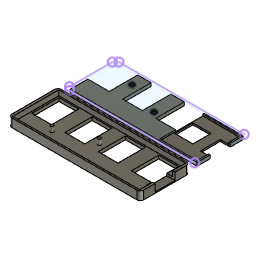
dongle_housing (Autodesk Fusion 360 design; units mm, degrees)
Autodesk Fusion 360 part; units mm, degrees
sketch "Sketch1" plane through (0, 0, 0) normal (0, 0, 1) x (1, 0, 0)
  line L0 (2, 0) -> (78, 0)
  line L1 (80, 2) -> (80, 28)
  line L2 (78, 30) -> (2, 30)
  line L3 (0, 28) -> (0, 2)
  arc A0 (2, 30) -> (0, 28) centre (2, 28) ccw
  arc A1 (0, 2) -> (2, 0) centre (2, 2) ccw
  arc A2 (80, 28) -> (78, 30) centre (78, 28) ccw
  arc A3 (78, 0) -> (80, 2) centre (78, 2) ccw
  point P0 (80, 0)
  point P1 (0, 30)
  dimension "d1" = 30
  dimension "d2" = 80
  dimension "d3" = 2
  dimension "d4" = 2
  dimension "d5" = 2
  dimension "d6" = 2
  constraint horizontal L0
  constraint vertical L1
  constraint horizontal L2
  constraint vertical L3
  constraint coincident P1 L2
  constraint coincident P1 L3
  constraint tangent L2 A0
  constraint tangent L3 A0
  constraint coincident origin L0
  constraint coincident origin L3
  constraint tangent L0 A1
  constraint tangent L3 A1
  constraint tangent L1 A2
  constraint tangent L2 A2
  constraint coincident P0 L0
  constraint coincident P0 L1
  constraint tangent L0 A3
  constraint tangent L1 A3
  measures "d1" distance of origin P1
  measures "d2" distance of origin P0
  measures "d3" radius of A0
  measures "d4" radius of A1
  measures "d5" radius of A2
  measures "d6" radius of A3
extrude "Extrude1" add sketch "Sketch1" along normal blind 6 makes body 1
sketch "Sketch2" plane through (0, 0, 6) normal (0, 0, 1) x (-1, 0, 0)
  arc A0 (-78, 0) -> (-80, -2) centre (-78, -2) ccw
  line L0 (-80, -2) -> (-80, -28)
  arc A1 (-80, -28) -> (-78, -30) centre (-78, -28) ccw
  line L1 (-78, -30) -> (-2, -30)
  arc A2 (-2, -30) -> (0, -28) centre (-2, -28) ccw
  line L2 (0, -28) -> (0, -2)
  arc A3 (0, -2) -> (-2, 0) centre (-2, -2) ccw
  line L3 (-2, 0) -> (-78, 0)
  line L4 (-40, -30) -> (-40, 0) construction
  line L5 (-2.5, -28.1) -> (-77.5, -28.1)
  line L6 (-77.5, -28.1) -> (-77.5, -1.9)
  line L7 (-77.5, -1.9) -> (-2.5, -1.9)
  line L8 (-2.5, -1.9) -> (-2.5, -28.1)
  line L9 (0, -15) -> (-80, -15) construction
  dimension "d11" = 75
  dimension "d12" = 26.2
  constraint midpoint L1 L4.start
  constraint midpoint L3 L4.end
  constraint horizontal L5
  constraint vertical L6
  constraint horizontal L7
  constraint vertical L8
  constraint symmetric L4 L6 L8
  constraint midpoint L2 L9.start
  constraint midpoint L0 L9.end
  constraint symmetric L5 L7 L9
  measures "d11" distance of L5.start L5.end
  measures "d12" distance of L5.end L6.end
extrude "Extrude2" cut sketch "Sketch2" against normal blind 4 contours L5 L6 L7 L8 bodies 1
sketch "Sketch4" plane through (0, 0, 6) normal (0, 0, 1) x (1, 0, 0)
  line L0 (2.5, 28.1) -> (14.5, 28.1)
  line L1 (14.5, 28.1) -> (14.5, 11.6)
  line L2 (14.5, 11.6) -> (2.5, 11.6)
  line L3 (2.5, 11.6) -> (2.5, 28.1)
  line L4 (34.6667, 28.1) -> (34.6667, 11.6)
  line L5 (22.6667, 28.1) -> (34.6667, 28.1)
  line L6 (22.6667, 11.6) -> (22.6667, 28.1)
  line L7 (34.6667, 11.6) -> (22.6667, 11.6)
  line L8 (54.8333, 28.1) -> (54.8333, 11.6)
  line L9 (42.8333, 28.1) -> (54.8333, 28.1)
  line L10 (42.8333, 11.6) -> (42.8333, 28.1)
  line L11 (54.8333, 11.6) -> (42.8333, 11.6)
  line L12 (75, 28.1) -> (75, 11.6)
  line L13 (63, 28.1) -> (75, 28.1)
  line L14 (63, 11.6) -> (63, 28.1)
  line L15 (75, 11.6) -> (63, 11.6)
  dimension "d23" = 16.5
  dimension "d24" = 12
  dimension "d27" = 60.5
  dimension "d28" = 0
  constraint horizontal L0
  constraint vertical L1
  constraint horizontal L2
  constraint vertical L3
  measures "d23" distance of L0.start L2.end
  measures "d24" distance of L0.start L0.end
extrude "Extrude4" cut sketch "Sketch4" against normal blind 11 bodies 1
sketch "Sketch5" plane through (0, 0, 6) normal (0, 0, 1) x (-1, 0, 0)
  line L0 (-77.5, -28.1) -> (-77.5, -1.9)
  line L1 (-77.5, -1.9) -> (-2.5, -1.9)
  line L2 (-2.5, -1.9) -> (-2.5, -28.1)
  line L3 (-2.5, -28.1) -> (-77.5, -28.1)
  arc A0 (-78, 0) -> (-80, -2) centre (-78, -2) ccw
  line L4 (-80, -2) -> (-80, -28)
  arc A1 (-80, -28) -> (-78, -30) centre (-78, -28) ccw
  line L5 (-78, -30) -> (-2, -30)
  arc A2 (-2, -30) -> (0, -28) centre (-2, -28) ccw
  line L6 (0, -28) -> (0, -2)
  arc A3 (0, -2) -> (-2, 0) centre (-2, -2) ccw
  line L7 (-2, 0) -> (-78, 0)
  line L8 (-80, -21.05) -> (-75, -21.05)
  line L9 (-75, -21.05) -> (-75, -8.95)
  line L10 (-75, -8.95) -> (-80, -8.95)
  line L11 (-80, -8.95) -> (-80, -21.05)
  line L12 (-80, -15) -> (0, -15) construction
  dimension "d31" = 12.1
  constraint horizontal L8
  constraint vertical L9
  constraint horizontal L10
  constraint vertical L11
  constraint coincident L4 L8.start
  constraint midpoint L4 L12.start
  constraint midpoint L6 L12.end
  constraint symmetric L8 L10 L12
  measures "d31" distance of L8.start L10.end
extrude "Extrude5" cut sketch "Sketch5" against normal blind 5.3 contours L0 L4 L8 L10 L11 | L0 L8 L9 L10 bodies 1
sketch "Sketch6" plane through (0, 0, 2) normal (0, 0, 1) x (-1, 0, 0)
  line L0 (-75, -8.95) -> (-75, -11.6)
  line L1 (-75, -11.6) -> (-63, -11.6)
  line L2 (-63, -11.6) -> (-63, -28.1)
  line L3 (-63, -28.1) -> (-54.8333, -28.1)
  line L4 (-54.8333, -28.1) -> (-54.8333, -11.6)
  line L5 (-54.8333, -11.6) -> (-42.8333, -11.6)
  line L6 (-42.8333, -11.6) -> (-42.8333, -28.1)
  line L7 (-42.8333, -28.1) -> (-34.6667, -28.1)
  line L8 (-34.6667, -28.1) -> (-34.6667, -11.6)
  line L9 (-34.6667, -11.6) -> (-22.6667, -11.6)
  line L10 (-22.6667, -11.6) -> (-22.6667, -28.1)
  line L11 (-22.6667, -28.1) -> (-14.5, -28.1)
  line L12 (-14.5, -28.1) -> (-14.5, -11.6)
  line L13 (-14.5, -11.6) -> (-2.5, -11.6)
  line L14 (-2.5, -11.6) -> (-2.5, -1.9)
  line L15 (-2.5, -1.9) -> (-77.5, -1.9)
  line L16 (-77.5, -1.9) -> (-77.5, -8.95)
  line L17 (-77.5, -8.95) -> (-75, -8.95)
  circle A0 centre (-18.17, -8.2) radius 0.95
  line L18 (-2, 0) -> (-78, 0)
  circle A1 centre (-39.2, -15.9) radius 0.95
  line L19 (-2.5, -1.9) -> (-2.5, -28.1)
  dimension "d34" = 15.67
  dimension "d35" = 8.2
  dimension "d36" = 1.9
  dimension "d37" = 12.2
  dimension "d38" = 36.7
  dimension "d39" = 1.9
  measures "d34" distance of L14 A0.centre
  measures "d35" distance of A0.centre L18
  measures "d36" diameter of A0
  measures "d37" distance of L7 A1.centre
  measures "d38" distance of A1.centre L19
  measures "d39" diameter of A1
extrude "Extrude6" add sketch "Sketch6" along normal blind 9.15 contours A0 | A1 bodies 1
sketch "Sketch7" plane through (0, 0, 0) normal (0, 0, 1) x (1, 0, 0)
  line L0 (2, 35) -> (78, 35)
  line L1 (80, 37) -> (80, 63)
  line L2 (78, 65) -> (2, 65)
  line L3 (0, 63) -> (0, 37)
  arc A0 (2, 65) -> (0, 63) centre (2, 63) ccw
  arc A1 (80, 63) -> (78, 65) centre (78, 63) ccw
  arc A2 (78, 35) -> (80, 37) centre (78, 37) ccw
  arc A3 (0, 37) -> (2, 35) centre (2, 37) ccw
  point P0 (0, 35)
  point P1 (80, 65)
  point P2 (0, 65)
  dimension "d42" = 30
  dimension "d43" = 80
  dimension "d44" = 2
  constraint horizontal L0
  constraint vertical L1
  constraint horizontal L2
  constraint vertical L3
  constraint coincident P2 L2
  constraint coincident P2 L3
  constraint tangent L2 A0
  constraint tangent L3 A0
  constraint coincident P1 L1
  constraint coincident P1 L2
  constraint tangent L1 A1
  constraint tangent L2 A1
  constraint equal A0 A1
  constraint tangent L0 A2
  constraint tangent L1 A2
  constraint equal A0 A2
  constraint coincident P0 L0
  constraint coincident P0 L3
  constraint tangent L0 A3
  constraint tangent L3 A3
  constraint equal A0 A3
  measures "d42" distance of P0 P2
  measures "d43" distance of P1 P2
  measures "d44" radius of A0
extrude "Extrude7" add sketch "Sketch7" along normal blind 4 separate body makes body 2
sketch "Sketch8" plane through (0, 0, 4) normal (0, 0, 1) x (-1, 0, 0)
  arc A0 (0, -37) -> (-2, -35) centre (-2, -37) ccw
  line L0 (-2, -35) -> (-78, -35)
  arc A1 (-78, -35) -> (-80, -37) centre (-78, -37) ccw
  line L1 (-80, -37) -> (-80, -63)
  arc A2 (-80, -63) -> (-78, -65) centre (-78, -63) ccw
  line L2 (-78, -65) -> (-2, -65)
  arc A3 (-2, -65) -> (0, -63) centre (-2, -63) ccw
  line L3 (0, -63) -> (0, -37)
  line L4 (-2.5, -36.9) -> (-77.5, -36.9)
  line L5 (-77.5, -36.9) -> (-77.5, -63.1)
  line L6 (-77.5, -63.1) -> (-2.5, -63.1)
  line L7 (-2.5, -63.1) -> (-2.5, -36.9)
  line L8 (-80, -50) -> (0, -50) construction
  line L9 (-40, -65) -> (-40, -35) construction
  dimension "d47" = 75
  dimension "d48" = 26.2
  dimension "d49" = 37.5
  dimension "d50" = 13.1
  constraint horizontal L4
  constraint vertical L5
  constraint horizontal L6
  constraint vertical L7
  constraint midpoint L1 L8.start
  constraint midpoint L3 L8.end
  constraint midpoint L2 L9.start
  constraint midpoint L0 L9.end
  measures "d47" distance of L5.end L6.end
  measures "d48" distance of L4 L6
  measures "d49" distance of L7 L9
  measures "d50" distance of L6 L8
extrude "Extrude8" cut sketch "Sketch8" against normal blind 2 contours L4 L5 L6 L7 bodies 2
sketch "Sketch9" plane through (0, 0, 2) normal (0, 0, 1) x (-1, 0, 0)
  line L0 (-2.5, -63.1) -> (-2.5, -36.9)
  line L1 (-2.5, -36.9) -> (-77.5, -36.9)
  line L2 (-77.5, -36.9) -> (-77.5, -63.1)
  line L3 (-77.5, -63.1) -> (-2.5, -63.1)
  line L4 (-2.5, -63.1) -> (-14.5, -63.1)
  line L5 (-14.5, -63.1) -> (-14.5, -46.6)
  line L6 (-14.5, -46.6) -> (-2.5, -46.6)
  line L7 (-2.5, -46.6) -> (-2.5, -63.1)
  line L8 (-34.65, -63.1) -> (-34.65, -46.6)
  line L9 (-22.65, -46.6) -> (-22.65, -63.1)
  line L10 (-34.65, -46.6) -> (-22.65, -46.6)
  line L11 (-22.65, -63.1) -> (-34.65, -63.1)
  line L12 (-54.8, -63.1) -> (-54.8, -46.6)
  line L13 (-42.8, -46.6) -> (-42.8, -63.1)
  line L14 (-54.8, -46.6) -> (-42.8, -46.6)
  line L15 (-42.8, -63.1) -> (-54.8, -63.1)
  dimension "d53" = 16.5
  dimension "d54" = 12
  dimension "d57" = -40.3
  dimension "d58" = 0
  constraint horizontal L4
  constraint vertical L5
  constraint horizontal L6
  constraint vertical L7
  constraint coincident L0.start L3.end
  measures "d53" distance of L0.start L6.end
  measures "d54" distance of L0.start L4.end
extrude "Extrude9" cut sketch "Sketch9" against normal blind 11 contours L0 L3 L4 L5 L6 L7 | L3 L8 L9 L10 L11 | L3 L12 L13 L14 L15 bodies 2
sketch "Sketch10" plane through (0, 0, 4) normal (0, 0, 1) x (-1, 0, 0)
  line L0 (-77.5, -36.9) -> (-2.5, -36.9)
  line L1 (-2.5, -36.9) -> (-2.5, -63.1)
  line L2 (-2.5, -63.1) -> (-77.5, -63.1)
  line L3 (-77.5, -63.1) -> (-77.5, -36.9)
  arc A0 (0, -37) -> (-2, -35) centre (-2, -37) ccw
  line L4 (-2, -35) -> (-78, -35)
  arc A1 (-78, -35) -> (-80, -37) centre (-78, -37) ccw
  line L5 (-80, -37) -> (-80, -63)
  arc A2 (-80, -63) -> (-78, -65) centre (-78, -63) ccw
  line L6 (-78, -65) -> (-2, -65)
  arc A3 (-2, -65) -> (0, -63) centre (-2, -63) ccw
  line L7 (0, -63) -> (0, -37)
  line L8 (-77.5, -43.95) -> (-83, -43.95)
  line L9 (-83, -43.95) -> (-83, -56.05)
  line L10 (-83, -56.05) -> (-77.5, -56.05)
  line L11 (-77.5, -56.05) -> (-77.5, -43.95)
  line L12 (-80, -50) -> (0, -50) construction
  line L13 (-77.5, -43.95) -> (-72.5, -43.95)
  line L14 (-72.5, -43.95) -> (-72.5, -56)
  line L15 (-72.5, -56) -> (-77.5, -56)
  line L16 (-77.5, -56) -> (-77.5, -43.95)
  dimension "d61" = 12.1
  dimension "d62" = 6.05
  dimension "d63" = 5
  constraint horizontal L8
  constraint vertical L9
  constraint horizontal L10
  constraint vertical L11
  constraint coincident L3 L8.start
  constraint midpoint L5 L12.start
  constraint midpoint L7 L12.end
  constraint horizontal L13
  constraint vertical L14
  constraint horizontal L15
  constraint vertical L16
  measures "d61" distance of L8.end L9.end
  measures "d62" distance of L10 L12
  measures "d63" distance of L8.start L13.end
extrude "Extrude10" cut sketch "Sketch10" against normal blind 2.5 contours L3 L11 L13 L14 L15 L16 | L3 L5 L8 L10 L11 L16 | L5 L8 L9 L10 bodies 2
sketch "Sketch11" plane through (0, 0, 2) normal (0, 0, 1) x (-1, 0, 0)
  line L0 (-72.5, -56) -> (-77.5, -56)
  line L1 (-77.5, -56) -> (-77.5, -56.05)
  line L2 (-77.5, -56.05) -> (-77.5, -63.1)
  line L3 (-77.5, -63.1) -> (-54.8, -63.1)
  line L4 (-54.8, -63.1) -> (-54.8, -46.6)
  line L5 (-54.8, -46.6) -> (-42.8, -46.6)
  line L6 (-42.8, -46.6) -> (-42.8, -63.1)
  line L7 (-42.8, -63.1) -> (-34.65, -63.1)
  line L8 (-34.65, -63.1) -> (-34.65, -46.6)
  line L9 (-34.65, -46.6) -> (-22.65, -46.6)
  line L10 (-22.65, -46.6) -> (-22.65, -63.1)
  line L11 (-22.65, -63.1) -> (-14.5, -63.1)
  line L12 (-14.5, -63.1) -> (-14.5, -46.6)
  line L13 (-14.5, -46.6) -> (-2.5, -46.6)
  line L14 (-2.5, -46.6) -> (-2.5, -36.9)
  line L15 (-2.5, -36.9) -> (-77.5, -36.9)
  line L16 (-77.5, -36.9) -> (-77.5, -43.95)
  line L17 (-77.5, -43.95) -> (-72.5, -43.95)
  line L18 (-72.5, -43.95) -> (-72.5, -56)
  line L19 (-77.5, -36.9) -> (-65.5, -36.9)
  line L20 (-65.5, -36.9) -> (-65.5, -63.1)
  line L21 (-65.5, -63.1) -> (-77.5, -63.1)
  line L22 (-77.5, -63.1) -> (-77.5, -36.9)
  dimension "d66" = 12
  constraint horizontal L19
  constraint vertical L20
  constraint horizontal L21
  constraint vertical L22
  constraint coincident L3 L20.end
  constraint coincident L15.end L16.start
  measures "d66" distance of L20 L22
extrude "Extrude11" cut sketch "Sketch11" against normal blind 1 contours L0 L1 L2 L3 L15 L16 L17 L18 L19 L20 L21 L22 bodies 2
sketch "Sketch12" plane through (0, 0, 2) normal (0, 0, 1) x (-1, 0, 0)
  line L0 (-65.5, -36.9) -> (-65.5, -63.1)
  line L1 (-65.5, -63.1) -> (-54.8, -63.1)
  line L2 (-54.8, -63.1) -> (-54.8, -46.6)
  line L3 (-54.8, -46.6) -> (-42.8, -46.6)
  line L4 (-42.8, -46.6) -> (-42.8, -63.1)
  line L5 (-42.8, -63.1) -> (-34.65, -63.1)
  line L6 (-34.65, -63.1) -> (-34.65, -46.6)
  line L7 (-34.65, -46.6) -> (-22.65, -46.6)
  line L8 (-22.65, -46.6) -> (-22.65, -63.1)
  line L9 (-22.65, -63.1) -> (-14.5, -63.1)
  line L10 (-14.5, -63.1) -> (-14.5, -46.6)
  line L11 (-14.5, -46.6) -> (-2.5, -46.6)
  line L12 (-2.5, -46.6) -> (-2.5, -36.9)
  line L13 (-2.5, -36.9) -> (-65.5, -36.9)
  line L14 (-55.5, -56.4) -> (-66.5, -56.4)
  line L15 (-66.5, -56.4) -> (-66.5, -45.4)
  line L16 (-66.5, -45.4) -> (-55.5, -45.4)
  line L17 (-55.5, -45.4) -> (-55.5, -56.4)
  line L18 (-77.5, -37) -> (-77.5, -63) construction
  dimension "d69" = 11
  dimension "d70" = 11
  dimension "d71" = 11
  dimension "d109" = 8.5
  constraint horizontal L14
  constraint vertical L15
  constraint horizontal L16
  constraint vertical L17
  constraint parallel L2 L18
  measures "d69" distance of L14.end L15.end
  measures "d70" distance of L14.start L14.end
  measures "d71" distance of L15 L18
  measures "d109" distance of L13 L16
extrude "Extrude12" cut sketch "Sketch12" against normal blind 8 contours L0 L14 L16 L17 | L0 L14 L15 L16 bodies 2
sketch "Sketch13" plane through (0, 0, 2) normal (0, 0, 1) x (-1, 0, 0)
  line L0 (-55.5, -56.4) -> (-65.5, -56.4)
  line L1 (-65.5, -56.4) -> (-65.5, -63.1)
  line L2 (-65.5, -63.1) -> (-54.8, -63.1)
  line L3 (-54.8, -63.1) -> (-54.8, -46.6)
  line L4 (-54.8, -46.6) -> (-42.8, -46.6)
  line L5 (-42.8, -46.6) -> (-42.8, -63.1)
  line L6 (-42.8, -63.1) -> (-34.65, -63.1)
  line L7 (-34.65, -63.1) -> (-34.65, -46.6)
  line L8 (-34.65, -46.6) -> (-22.65, -46.6)
  line L9 (-22.65, -46.6) -> (-22.65, -63.1)
  line L10 (-22.65, -63.1) -> (-14.5, -63.1)
  line L11 (-14.5, -63.1) -> (-14.5, -46.6)
  line L12 (-14.5, -46.6) -> (-2.5, -46.6)
  line L13 (-2.5, -46.6) -> (-2.5, -36.9)
  line L14 (-2.5, -36.9) -> (-65.5, -36.9)
  line L15 (-65.5, -36.9) -> (-65.5, -45.4)
  line L16 (-65.5, -45.4) -> (-55.5, -45.4)
  line L17 (-55.5, -45.4) -> (-55.5, -56.4)
  line L18 (-54.8, -63.1) -> (-65.5, -63.1)
  line L19 (-65.5, -63.1) -> (-65.5, -36.9)
  line L20 (-65.5, -36.9) -> (-54.8, -36.9)
  line L21 (-54.8, -36.9) -> (-54.8, -63.1)
  constraint horizontal L18
  constraint vertical L19
  constraint horizontal L20
  constraint vertical L21
  constraint coincident L14.end L15.start
  constraint coincident L2.end L3.start
extrude "Extrude13" cut sketch "Sketch13" against normal blind 1 contours L0 L1 L2 L3 L14 L15 L16 L17 L18 L19 L20 L21 bodies 2
sketch "Sketch14" plane through (0, 0, 6) normal (0, 0, 1) x (-1, 0, 0)
  line L0 (-77.5, -21.05) -> (-80, -21.05)
  line L1 (-80, -21.05) -> (-80, -28)
  arc A0 (-80, -28) -> (-78, -30) centre (-78, -28) ccw
  line L2 (-78, -30) -> (-2, -30)
  arc A1 (-2, -30) -> (0, -28) centre (-2, -28) ccw
  line L3 (0, -28) -> (0, -2)
  arc A2 (0, -2) -> (-2, 0) centre (-2, -2) ccw
  line L4 (-2, 0) -> (-78, 0)
  arc A3 (-78, 0) -> (-80, -2) centre (-78, -2) ccw
  line L5 (-80, -2) -> (-80, -8.95)
  line L6 (-80, -8.95) -> (-77.5, -8.95)
  line L7 (-77.5, -8.95) -> (-77.5, -1.9)
  line L8 (-77.5, -1.9) -> (-2.5, -1.9)
  line L9 (-2.5, -1.9) -> (-2.5, -28.1)
  line L10 (-2.5, -28.1) -> (-77.5, -28.1)
  line L11 (-77.5, -28.1) -> (-77.5, -21.05)
  line L12 (-1.5, -1) -> (-78.5, -1)
  line L13 (-78.5, -1) -> (-78.5, -29)
  line L14 (-78.5, -29) -> (-1.5, -29)
  line L15 (-1.5, -29) -> (-1.5, -1)
  dimension "d77" = 77
  dimension "d78" = 28
  dimension "d79" = 1
  dimension "d80" = 1.5
  constraint horizontal L12
  constraint vertical L13
  constraint horizontal L14
  constraint vertical L15
  measures "d77" distance of L12.start L12.end
  measures "d78" distance of L12.start L14.end
  measures "d79" distance of L4 L12
  measures "d80" distance of L3 L15
extrude "Extrude14" cut sketch "Sketch14" against normal blind 2.87 contours L0 L6 L7 L8 L9 L10 L11 L12 L13 L14 L15 bodies 1
sketch "Sketch15" plane through (0, 0, 4) normal (0, 0, 1) x (-1, 0, 0)
  line L0 (-77.5, -56.05) -> (-80, -56.05)
  line L1 (-80, -56.05) -> (-80, -63)
  arc A0 (-80, -63) -> (-78, -65) centre (-78, -63) ccw
  line L2 (-78, -65) -> (-2, -65)
  arc A1 (-2, -65) -> (0, -63) centre (-2, -63) ccw
  line L3 (0, -63) -> (0, -37)
  arc A2 (0, -37) -> (-2, -35) centre (-2, -37) ccw
  line L4 (-2, -35) -> (-78, -35)
  arc A3 (-78, -35) -> (-80, -37) centre (-78, -37) ccw
  line L5 (-80, -37) -> (-80, -43.95)
  line L6 (-80, -43.95) -> (-77.5, -43.95)
  line L7 (-77.5, -43.95) -> (-77.5, -36.9)
  line L8 (-77.5, -36.9) -> (-2.5, -36.9)
  line L9 (-2.5, -36.9) -> (-2.5, -63.1)
  line L10 (-2.5, -63.1) -> (-77.5, -63.1)
  line L11 (-77.5, -63.1) -> (-77.5, -56.05)
  line L12 (-1.5, -35.9) -> (-78.5, -35.9)
  line L13 (-78.5, -35.9) -> (-78.5, -63.9)
  line L14 (-78.5, -63.9) -> (-1.5, -63.9)
  line L15 (-1.5, -63.9) -> (-1.5, -35.9)
  dimension "d83" = 77
  dimension "d84" = 28
  dimension "d85" = 1
  dimension "d86" = 1
  constraint horizontal L12
  constraint vertical L13
  constraint horizontal L14
  constraint vertical L15
  measures "d83" distance of L13.end L14.end
  measures "d84" distance of L12.start L14.end
  measures "d85" distance of L9 L15
  measures "d86" distance of L8 L12
extrude "Extrude15" cut sketch "Sketch15" against normal blind 2 contours L0 L1 A0 L2 A1 L3 A2 L4 A3 L5 L6 L12 L13 L14 L15 bodies 2
extrude "Extrude16" cut 1 faces at (27.5, 36.2333, 4) along direction (0, 0, -1) blind 2 on bodies 2 bodies 2
extrude "Extrude17" cut 1 faces at (1, 19.3333, 6) along direction (0, 0, -1) up to surface (0.87 mm away) on bodies 1 bodies 1
sketch "Sketch16" plane through (0, 0, 2) normal (0, 0, 1) x (-1, 0, 0)
  line L0 (-14.5, -63.1) -> (-14.5, -46.6)
  line L1 (-14.5, -46.6) -> (-2.5, -46.6)
  line L2 (-2.5, -46.6) -> (-2.5, -63.1)
  line L3 (-2.5, -63.1) -> (-14.5, -63.1)
  line L4 (-54.8, -36.9) -> (-54.8, -46.6)
  line L5 (-54.8, -46.6) -> (-42.8, -46.6)
  line L6 (-42.8, -46.6) -> (-42.8, -63.1)
  line L7 (-42.8, -63.1) -> (-77.5, -63.1)
  line L8 (-77.5, -63.1) -> (-77.5, -56.05)
  line L9 (-77.5, -56.05) -> (-80, -56.05)
  line L10 (-80, -56.05) -> (-80, -63)
  arc A0 (-80, -63) -> (-78, -65) centre (-78, -63) ccw
  line L11 (-78, -65) -> (-2, -65)
  arc A1 (-2, -65) -> (0, -63) centre (-2, -63) ccw
  line L12 (0, -63) -> (0, -37)
  arc A2 (0, -37) -> (-2, -35) centre (-2, -37) ccw
  line L13 (-2, -35) -> (-78, -35)
  arc A3 (-78, -35) -> (-80, -37) centre (-78, -37) ccw
  line L14 (-80, -37) -> (-80, -43.95)
  line L15 (-80, -43.95) -> (-77.5, -43.95)
  line L16 (-77.5, -43.95) -> (-77.5, -36.9)
  line L17 (-77.5, -36.9) -> (-54.8, -36.9)
  line L18 (-22.65, -63.1) -> (-34.65, -63.1)
  line L19 (-34.65, -63.1) -> (-34.65, -46.6)
  line L20 (-34.65, -46.6) -> (-22.65, -46.6)
  line L21 (-22.65, -46.6) -> (-22.65, -63.1)
  circle A4 centre (-39.2, -49.1) radius 1.175
  circle A5 centre (-18.17, -56.8) radius 1.175
  line L22 (-2, -35) -> (-78, -35)
  line L23 (0, -63) -> (0, -37)
  line L24 (-78, -65) -> (-2, -65)
  dimension "d93" = 2.35
  dimension "d94" = 2.35
  dimension "d95" = 14.1
  dimension "d96" = 39.2
  dimension "d97" = 18.17
  dimension "d98" = 8.2
  measures "d93" diameter of A4
  measures "d94" diameter of A5
  measures "d95" distance of A4.centre L22
  measures "d96" distance of A4.centre L23
  measures "d97" distance of A5.centre L23
  measures "d98" distance of A5.centre L24
extrude "Extrude18" cut sketch "Sketch16" against normal blind 5 contours A4 | A5 bodies 2
extrude "Extrude19" cut sketch "Sketch15" against normal blind 23 contours L0 L1 A0 L2 A1 L3 A2 L4 A3 L5 L6 L12 L13 L14 L15 bodies 2
extrude "Extrude20" cut 2 faces at (17.8674, 8.2933, 11.15) (39.3974, 16.242, 11.15) along direction (0, 0, 1) up to surface end surface through (0, 0, 5.13) normal (0, 0, 1) offset 0 on bodies 1 bodies 1
extrude "Extrude21" cut 1 faces at (74.1667, 51.9833, 1.5) along direction (0, 0, -1) blind 15 on bodies 2 bodies 2
extrude "Extrude22" cut 1 faces at (1.8333, 19.3667, 3.13) along direction (0, 0, -1) up to surface (1.13 mm away) on bodies 1 bodies 1
sketch "Sketch17" plane through (0, 0, 2) normal (0, 0, 1) x (-1, 0, 0)
  line L0 (-78.5, -35.9) -> (-78.5, -43.95)
  line L1 (-78.5, -43.95) -> (-77.5, -43.95)
  line L2 (-77.5, -43.95) -> (-77.5, -36.9)
  line L3 (-77.5, -36.9) -> (-54.8, -36.9)
  line L4 (-54.8, -36.9) -> (-54.8, -46.6)
  line L5 (-54.8, -46.6) -> (-42.8, -46.6)
  line L6 (-42.8, -46.6) -> (-42.8, -63.1)
  line L7 (-42.8, -63.1) -> (-77.5, -63.1)
  line L8 (-77.5, -63.1) -> (-77.5, -56.05)
  line L9 (-77.5, -56.05) -> (-78.5, -56.05)
  line L10 (-78.5, -56.05) -> (-78.5, -63.9)
  line L11 (-78.5, -63.9) -> (-1.5, -63.9)
  line L12 (-1.5, -63.9) -> (-1.5, -35.9)
  line L13 (-1.5, -35.9) -> (-78.5, -35.9)
  circle A0 centre (-18.17, -56.8) radius 1.175
  circle A1 centre (-39.2, -49.1) radius 1.175
  line L14 (-14.5, -63.1) -> (-14.5, -46.6)
  line L15 (-14.5, -46.6) -> (-2.5, -46.6)
  line L16 (-2.5, -46.6) -> (-2.5, -63.1)
  line L17 (-2.5, -63.1) -> (-14.5, -63.1)
  line L18 (-22.65, -63.1) -> (-34.65, -63.1)
  line L19 (-34.65, -63.1) -> (-34.65, -46.6)
  line L20 (-34.65, -46.6) -> (-22.65, -46.6)
  line L21 (-22.65, -46.6) -> (-22.65, -63.1)
  line L22 (-14.5, -46.6) -> (-1.5, -46.6)
  line L23 (-1.5, -46.6) -> (-1.5, -63.9)
  line L24 (-1.5, -63.9) -> (-14.5, -63.9)
  line L25 (-14.5, -63.9) -> (-14.5, -46.6)
  line L26 (-34.65, -46.6) -> (-22.65, -46.6)
  line L27 (-22.65, -46.6) -> (-22.65, -63.9)
  line L28 (-22.65, -63.9) -> (-34.65, -63.9)
  line L29 (-34.65, -63.9) -> (-34.65, -46.6)
  line L30 (-42.8, -46.6) -> (-54.8, -46.6)
  line L31 (-54.8, -46.6) -> (-54.8, -63.9)
  line L32 (-54.8, -63.9) -> (-42.8, -63.9)
  line L33 (-42.8, -63.9) -> (-42.8, -46.6)
  constraint horizontal L22
  constraint vertical L23
  constraint horizontal L24
  constraint vertical L25
  constraint coincident L11.end L12.start
  constraint coincident L14.end L15.start
  constraint horizontal L26
  constraint vertical L27
  constraint horizontal L28
  constraint vertical L29
  constraint coincident L11 L27.end
  constraint coincident L19.end L20.start
  constraint horizontal L30
  constraint vertical L31
  constraint horizontal L32
  constraint vertical L33
  constraint coincident L11 L31.end
  constraint coincident L5.end L6.start
extrude "Extrude23" cut sketch "Sketch17" against normal blind 11 contours L11 L12 L16 L17 L22 L23 L24 L25 | L11 L18 L27 L28 L29 | L7 L11 L31 L32 L33 bodies 2
extrude "Extrude3" [suppressed]
equation "d32 = -4.00 mm - 1.3 mm"
equation "d35 = 6.7 mm + 1.5 mm"
equation "d49 = ( 75 / 2 ) * 1 mm"
equation "d50 = ( 26.2 / 2 ) * 1 mm"
equation "d62 = ( 12.1 / 2 ) * 1 mm"
equation "d81 = -4.00 mm + 1.13 mm"
equation "d95 = 12.2 mm + 1.9 mm"
equation "d96 = 36.7 mm + 2.5 mm"
equation "d97 = 15.67 mm + 2.5 mm"
equation "d98 = 6.7 mm + 1.5 mm"
